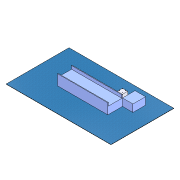
# Autodesk Inventor part: Environment
Saved by Autodesk Inventor 2021 (Build 250183000, 183)
## iProperties
Created: 2021-04-02
Part Number: Environment
Material: Generic
Document SubType Name: Modeling
Designer: Tran Duc Viet
Mass: 895857 g
Surface Area: 391453 cm^2
Volume: 895857 cm^3
Density: 1 g/cm^3
Appearance: Default
Author: Tran Duc Viet
Autodesk Inventor part; units mm, degrees
ref_plane "YZ Plane" through (0, 0, 0) normal (1, 0, 0) x (0, 1, 0)
ref_plane "XZ Plane" through (0, 0, 0) normal (0, 1, 0) x (-1, 0, 0)
ref_plane "XY Plane" through (0, 0, 0) normal (0, 0, 1) x (1, 0, 0)
sketch "Sketch1" plane through (0, 0, 0) normal (0, 1, 0) x (-1, 0, 0)
  line L0 (1200, 350) -> (-1200, 350)
  line L1 (-1200, 350) -> (-1200, -350)
  line L2 (-1200, -350) -> (1200, -350)
  line L3 (1200, -350) -> (1200, 350)
  line L4 (1200, 350) -> (-1200, -350) construction
  line L5 (-1200, 350) -> (1200, -350) construction
  point P0 (0, 0)
  dimension "d0" = 2400
  dimension "d1" = 700
  constraints: 12 end point, 2 midpoint, 2 parallel, 1 horizontal, 1 perpendicular
  measures "d0" distance of L2.end L1.end
  measures "d1" distance of L1.end L0.end
extrude "Extrusion1" add sketch "Sketch1" along normal blind 500
sketch "Sketch2" plane through (0, 500, 0) normal (0, 1, 0) x (1, 0, 0)
  line L0 (1200, -350) -> (1200, 350) projected
  line L1 (1200, 350) -> (950, 350)
  line L2 (950, 350) -> (950, 600)
  line L3 (950, 600) -> (1200, 600)
  line L4 (1200, 600) -> (1200, 350)
  point P0 (0, 0)
  dimension "d4" = 250
  dimension "d5" = 250
  constraints: 8 end point, 2 parallel, 1 horizontal, 1 perpendicular
  measures "d4" distance of L2.end L3.end
  measures "d5" distance of L1.end L2.end
extrude "Extrusion2" add sketch "Sketch2" against normal blind 500
sketch "Sketch3" plane through (0, 500, 0) normal (0, 1, 0) x (1, 0, 0)
  line L0 (975, 575) -> (1125, 575)
  line L1 (1125, 575) -> (1125, 425)
  line L2 (1125, 425) -> (975, 425)
  line L3 (975, 425) -> (975, 575)
  line L4 (1200, 600) -> (950, 600) projected
  line L5 (950, 600) -> (950, 350) projected
  circle A0 centre (975, 575) radius 6
  circle A1 centre (1125, 575) radius 6
  circle A2 centre (975, 425) radius 6
  circle A3 centre (1125, 425) radius 6
  point P0 (0, 0)
  dimension "d16" = 150
  dimension "d17" = 150
  dimension "d18" = 25
  dimension "d19" = 25
  dimension "d20" = 12
  dimension "d21" = 12
  dimension "d22" = 12
  dimension "d23" = 12
  constraints: 8 end point, 4 centre point, 4 coincident, 2 parallel, 1 horizontal, 1 perpendicular
  measures "d16" distance of L0.start L0.end
  measures "d17" distance between parallel lines of L2 L0
  measures "d18" distance between parallel lines of L4 L0
  measures "d19" distance between parallel lines of L5 L3
  measures "d20" diameter of A0
  measures "d21" diameter of A1
  measures "d22" diameter of A2
  measures "d23" diameter of A3
extrude "Extrusion3" add sketch "Sketch3" along normal blind 15 contours L3 A0 L0 | L0 A0 L3 | A1 L1 L0 | L0 L1 A1 | A2 L2 L3 | L3 L2 A2 | A3 L2 L1 | L1 L2 A3
sketch "Sketch4" plane through (0, 500, 0) normal (0, 1, 0) x (1, 0, 0)
  line L0 (1200, -350) -> (1200, 600) projected
  line L1 (1200, 350) -> (1700, 350)
  line L2 (1700, 350) -> (1700, 950)
  line L3 (1700, 950) -> (1200, 950)
  line L4 (1200, 950) -> (1200, 350)
  line L5 (1200, 600) -> (950, 600) projected
  point P0 (0, 0)
  dimension "d26" = 500
  dimension "d27" = 600
  dimension "d28" = 250
  constraints: 8 end point, 2 parallel, 1 horizontal, 1 perpendicular, 1 point on line
  measures "d26" distance of L3.end L2.end
  measures "d27" distance of L2.end L1.end
  measures "d28" distance between parallel lines of L1 L5
extrude "Extrusion4" add sketch "Sketch4" against normal blind 500
sketch "Sketch7" plane through (1200, 0, 350) normal (1, 0, 0) x (0, 0, -1)
  line L0 (0, 500) -> (700, 500) projected
  line L1 (30, 500) -> (670, 500)
  line L2 (670, 500) -> (670, 350)
  line L3 (670, 350) -> (30, 350)
  line L4 (30, 350) -> (30, 500)
  line L5 (0, 0) -> (0, 500) projected
  point P0 (350, 0)
  dimension "d45" = 640
  dimension "d46" = 150
  dimension "d47" = 30
  constraints: 8 end point, 2 parallel, 1 horizontal, 1 perpendicular, 1 point on line
  measures "d45" distance of L2.end L3.end
  measures "d46" distance of L1.end L2.end
  measures "d47" distance between parallel lines of L5 L4
extrude "Extrusion5" cut sketch "Sketch7" against normal up to next
sketch "Sketch8" plane through (0, 0, 0) normal (0, -1, 0) x (1, 0, 0)
  line L0 (-2500, -1500) -> (2500, -1500)
  line L1 (2500, -1500) -> (2500, 1500)
  line L2 (2500, 1500) -> (-2500, 1500)
  line L3 (-2500, 1500) -> (-2500, -1500)
  line L4 (-2500, -1500) -> (2500, 1500) construction
  line L5 (2500, -1500) -> (-2500, 1500) construction
  point P0 (0, 0)
  dimension "d50" = 5000
  dimension "d51" = 3000
  constraints: 12 end point, 2 midpoint, 2 parallel, 1 horizontal, 1 perpendicular
  measures "d50" distance of L2.end L1.end
  measures "d51" distance of L1.end L0.end
extrude "Extrusion6" add sketch "Sketch8" along normal blind 10
split body "Split1" result two bodies by plane through (0, 0, 0) normal (0, 1, 0) first body at (316.6667, 0.5, 116.6667)
ref_plane "Work Plane2" through (1200, 500, -350) normal (0, 0, 1) x (1, 0, 0)
split body "Split2" result two bodies by plane through (1200, 500, -350) normal (0, 0, 1) bodies 2 first body at (316.6667, 0.5, 116.6667)
sketch "Sketch9" plane through (0, 500, 0) normal (0, 1, 0) x (1, 0, 0)
  line L0 (1700, 950) -> (1200, 950)
  line L1 (1200, 950) -> (1200, 350)
  line L2 (1200, 350) -> (1700, 350)
  line L3 (1700, 350) -> (1700, 950)
  point P0 (0, 0)
  constraints: 8 end point, 2 parallel, 1 horizontal, 1 perpendicular
extrude "Extrusion7" cut sketch "Sketch9" against normal blind 150 bodies 5
ref_plane "Work Plane3" through (1200, 350, -320) normal (1, 0, 0) x (0, 0, -1)
split body "Split4" result two bodies by plane through (1200, 350, -320) normal (1, 0, 0) bodies 5 first body at (1533.3333, 0.5, -633.3333)
